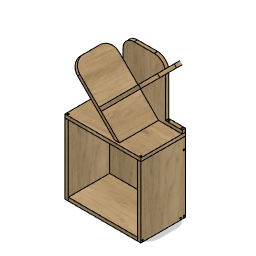
Project 02 Draft 1 (Autodesk Fusion 360 design; units mm, degrees)
Autodesk Fusion 360 part; units mm, degrees
sketch "Sketch1" plane through (0, 0, 0) normal (0, 1, 0) x (1, 0, 0)
  line L0 (0, 0) -> (340, 0)
  line L1 (340, 0) -> (340, -200)
  line L2 (340, -200) -> (0, -200)
  line L3 (0, -200) -> (0, 0)
  line L4 (0, 0) -> (15, 0)
  line L5 (15, 0) -> (15, -200)
  line L6 (15, -200) -> (0, -200)
  line L7 (0, -200) -> (0, 0)
  line L8 (340, 0) -> (325, 0)
  line L9 (325, 0) -> (325, -200)
  line L10 (325, -200) -> (340, -200)
  line L11 (340, -200) -> (340, 0)
  line L12 (15, 0) -> (325, 0)
  line L13 (325, 0) -> (325, -15)
  line L14 (325, -15) -> (15, -15)
  line L15 (15, -15) -> (15, 0)
  dimension "d1" = 340
  dimension "d2" = 200
  dimension "d3" = 15
  dimension "d4" = 15
  dimension "d5" = 15
  constraint horizontal L0
  constraint vertical L1
  constraint horizontal L2
  constraint vertical L3
  constraint coincident L0.start L3.end
  constraint horizontal L4
  constraint vertical L5
  constraint horizontal L6
  constraint vertical L7
  constraint coincident L2 L5.end
  constraint horizontal L8
  constraint vertical L9
  constraint horizontal L10
  constraint vertical L11
  constraint coincident L2 L9.end
  constraint horizontal L12
  constraint vertical L13
  constraint horizontal L14
  constraint vertical L15
  constraint coincident L9 L13.end
  measures "d1" distance of L0.start L0.end
  measures "d2" distance of L0.start L2.end
  measures "d3" distance of L0.start L4.end
  measures "d4" distance of L0.end L8.end
  measures "d5" distance of L4.end L14.end
extrude "Extrude1" add sketch "Sketch1" along normal blind 540 contours L0 L5 L9 L12 L13 L14 L15 makes body 1
extrude "Extrude2" add sketch "Sketch1" along normal blind 540 separate body contours L0 L2 L3 L4 L5 L6 L7 L15 makes body 2
extrude "Extrude3" add sketch "Sketch1" along normal blind 540 separate body contours L0 L1 L2 L8 L9 L10 L11 L13 makes body 3
sketch "Sketch2" plane through (15, 0, 0) normal (1, 0, 0) x (0, 0, -1)
  line L0 (-200, 0) -> (0, 0)
  line L1 (0, 0) -> (0, 540)
  line L2 (0, 540) -> (-200, 540)
  line L3 (-200, 540) -> (-200, 0)
  line L4 (-15, 225) -> (-200, 225)
  line L5 (-200, 225) -> (-200, 240)
  line L6 (-200, 240) -> (-15, 240)
  line L7 (-15, 240) -> (-15, 225)
  dimension "d14" = 15
  constraint horizontal L4
  constraint vertical L5
  constraint horizontal L6
  constraint vertical L7
  constraint coincident L3 L5.end
  measures "d14" distance of L4.start L6.end
extrude "Extrude5" add sketch "Sketch2" along normal blind 310 separate body contours L3 L4 L5 L6 L7 makes body 4
sketch "Sketch3" plane through (0, 540, 0) normal (0, 1, 0) x (-1, 0, 0)
  line L0 (-15, 200) -> (-15, 0)
  line L1 (-15, 0) -> (0, 0)
  line L2 (0, 0) -> (0, 200)
  line L3 (0, 200) -> (-15, 200)
  line L4 (0, 0) -> (-340, 0)
  line L5 (-340, 0) -> (-340, 200)
  line L6 (-340, 200) -> (0, 200)
  line L7 (0, 200) -> (0, 0)
  constraint horizontal L4
  constraint vertical L5
  constraint horizontal L6
  constraint vertical L7
  constraint coincident L1.end L2.start
extrude "Extrude6" add sketch "Sketch3" along normal blind 15 separate body makes body 5
sketch "Sketch4" plane through (0, 555, 0) normal (0, 1, 0) x (-1, 0, 0)
  line L0 (0, 200) -> (-340, 200)
  line L1 (-340, 200) -> (-340, 0)
  line L2 (-340, 0) -> (0, 0)
  line L3 (0, 0) -> (0, 200)
  line L4 (-75, 0) -> (-265, 0)
  line L5 (-265, 0) -> (-265, 15)
  line L6 (-265, 15) -> (-75, 15)
  line L7 (-75, 15) -> (-75, 0)
  dimension "d19" = 15
  constraint horizontal L4
  constraint vertical L5
  constraint horizontal L6
  constraint vertical L7
  constraint coincident L2 L4.start
  measures "d19" distance of L4.start L6.end
extrude "Extrude7" add sketch "Sketch4" along normal blind 250 separate body contours L2 L4 L5 L6 L7 makes body 6
sketch "Sketch5" plane through (0, 0, 15) normal (0, 0, 1) x (1, 0, 0)
  line L0 (75, 555) -> (265, 555)
  line L1 (265, 555) -> (265, 805)
  line L2 (265, 805) -> (75, 805)
  line L3 (75, 805) -> (75, 555)
  line L4 (0, 555) -> (170, 555) construction
  line L5 (170, 555) -> (234, 555) construction
  line L6 (234, 555) -> (21.868, 767.132)
  line L7 (234, 555) -> (494, 555) construction
  line L8 (21.868, 767.132) -> (11.2614, 756.5254)
  line L9 (11.2614, 756.5254) -> (212.7868, 555)
  line L10 (11.2614, 756.5254) -> (284.5456, 756.5254) construction
  line L11 (234, 555) -> (152.6827, 636.3173) construction
  line L12 (152.6827, 636.3173) -> (364.8148, 848.4493)
  line L13 (364.8148, 848.4493) -> (354.2082, 859.0559)
  line L14 (354.2082, 859.0559) -> (142.0761, 646.9239)
  dimension "d22" = 64
  dimension "d23" = 135
  dimension "d24" = 300
  dimension "d25" = 15
  dimension "d26" = 45
  dimension "d27" = 115
  dimension "d28" = 90
  dimension "d29" = 300
  dimension "d30" = 15
  constraint midpoint L0 L4.end
  constraint parallel L0 L4
  constraint coincident L0 L5.end
  constraint horizontal L7
  constraint perpendicular L6 L8
  constraint horizontal L10
  constraint coincident L5 L9.end
  constraint coincident L6 L11.end
  constraint perpendicular L12 L13
  constraint coincident L6 L14.end
  constraint perpendicular L6 L14
  measures "d22" distance of L4.end L5.end
  measures "d23" angle of L6 L7
  measures "d24" distance of L5.end L6.end
  measures "d25" distance of L6.end L8.end
  measures "d26" angle of L9 L10
  measures "d27" distance of L5.end L11.end
  measures "d28" angle of L11 L12
  measures "d29" distance of L11.end L12.end
  measures "d30" distance of L12.end L13.end
extrude "Extrude8" add sketch "Sketch5" along normal blind 175 separate body contours L0 L3 L6 L9 | L3 L6 L8 L9 makes body 7
extrude "Extrude9" add sketch "Sketch5" along normal blind 175 separate body contours L1 L6 L12 L14 | L1 L12 L13 L14 makes body 8
fillet "Fillet1" radius 50 2 edges at (265, 805, 7.5) (75, 805, 7.5) on bodies 6
fillet "Fillet2" radius 50 4 edges at (16.5647, 761.8287, 190) (16.5647, 761.8287, 15) (359.5115, 853.7526, 190) (359.5115, 853.7526, 15) on bodies 7 8
extrude "Extrude10" add 2 faces at (5, 0, 71.6667) (335, 0, 71.6667) along direction (0, -1, 0) blind 90 on bodies 2 3 bodies 2 3 4 5 6 7 8
extrude "Extrude11" add 1 faces at (118.3333, 0, 5) along direction (0, -1, 0) blind 90 on bodies 1 bodies 1
move_body "Move1" bodies 2 3 7 4 5 6 8 1 to x (1, 0, 0) y (0, 1, 0) z (0, 0, 1) at (0, 90, 0)
extrude "Extrude13" cut 1 faces at (118.3333, 0, 5) along direction (0, 1, 0) blind 315 on bodies 1 bodies 1
extrude "Extrude14" cut 1 faces at (5, 0, 66.6667) along direction (0, 1, 0) blind 315 on bodies 2 bodies 2
extrude "Extrude15" cut 1 faces at (330, 0, 66.6667) along direction (0, 1, 0) blind 315 on bodies 3 bodies 3
move_body "Move2" bodies 1 2 5 8 7 6 3 4 to x (1, 0, 0) y (0, 1, 0) z (0, 0, 1) at (0, -315, 0)
sketch "Sketch10" plane through (0, 315, 0) normal (0, 1, 0) x (-1, 0, 0)
  line L0 (-15, 200) -> (-15, 0)
  line L1 (-15, 0) -> (0, 0)
  line L2 (0, 0) -> (0, 200)
  line L3 (0, 200) -> (-15, 200)
  line L4 (0, 0) -> (-7.5, 0) construction
  line L5 (-7.5, 0) -> (-7.5, 7.5) construction
  line L6 (-7.5, 7.5) -> (0, 7.5) construction
  line L7 (0, 7.5) -> (0, 0) construction
  line L8 (0, 200) -> (-7.5, 200) construction
  line L9 (-7.5, 200) -> (-7.5, 192.5) construction
  line L10 (-7.5, 192.5) -> (0, 192.5) construction
  line L11 (0, 192.5) -> (0, 200) construction
  line L12 (-340, 200) -> (-332.5, 200) construction
  line L13 (-332.5, 200) -> (-332.5, 192.5) construction
  line L14 (-332.5, 192.5) -> (-340, 192.5) construction
  line L15 (-340, 192.5) -> (-340, 200) construction
  line L16 (-340, 0) -> (-332.5, 0) construction
  line L17 (-332.5, 0) -> (-332.5, 7.5) construction
  line L18 (-332.5, 7.5) -> (-340, 7.5) construction
  line L19 (-340, 7.5) -> (-340, 0) construction
  circle A0 centre (-7.5, 7.5) radius 4
  circle A1 centre (-7.5, 192.5) radius 4
  circle A2 centre (-332.5, 192.5) radius 4
  circle A3 centre (-332.5, 7.5) radius 4
  dimension "d66" = 7.5
  dimension "d67" = 7.5
  dimension "d68" = 7.5
  dimension "d69" = 7.5
  dimension "d70" = 7.5
  dimension "d71" = 7.5
  dimension "d72" = 7.5
  dimension "d73" = 7.5
  dimension "d74" = 8
  dimension "d75" = 8
  dimension "d76" = 8
  dimension "d77" = 8
  constraint horizontal L4
  constraint vertical L5
  constraint horizontal L6
  constraint vertical L7
  constraint coincident L1.end L2.start
  constraint horizontal L8
  constraint vertical L9
  constraint horizontal L10
  constraint vertical L11
  constraint coincident L2.end L3.start
  constraint horizontal L12
  constraint vertical L13
  constraint horizontal L14
  constraint vertical L15
  constraint horizontal L16
  constraint vertical L17
  constraint horizontal L18
  constraint vertical L19
  constraint coincident L5.end L6.start
  constraint coincident L9.end L10.start
  constraint coincident L13.end L14.start
  constraint coincident L17.end L18.start
  measures "d66" distance of L1.end L4.end
  measures "d67" distance of L1.end L6.end
  measures "d68" distance of L2.end L8.end
  measures "d69" distance of L2.end L10.end
  measures "d70" distance of L12.start L12.end
  measures "d71" distance of L12.start L14.end
  measures "d72" distance of L16.start L16.end
  measures "d73" distance of L16.start L18.end
  measures "d74" diameter of A0
  measures "d75" diameter of A1
  measures "d76" diameter of A2
  measures "d77" diameter of A3
sketch "Sketch11" plane through (265, 0, 0) normal (1, 0, 0) x (0, 0, -1)
  line L0 (0, 530) -> (-15, 530)
  line L1 (-15, 530) -> (-15, 330)
  line L2 (-15, 330) -> (0, 330)
  line L3 (0, 330) -> (0, 530)
  line L4 (-15, 330) -> (0, 330)
  line L5 (0, 330) -> (0, 345)
  line L6 (0, 345) -> (-15, 345)
  line L7 (-15, 345) -> (-15, 330)
  dimension "d78" = 15
  constraint horizontal L4
  constraint vertical L5
  constraint horizontal L6
  constraint vertical L7
  constraint coincident L1.end L2.start
  measures "d78" distance of L1.end L6.end
sketch "Sketch12" plane through (75, 0, 0) normal (-1, 0, 0) x (0, 0, 1)
  line L0 (15, 530) -> (0, 530)
  line L1 (0, 530) -> (0, 330)
  line L2 (0, 330) -> (15, 330)
  line L3 (15, 330) -> (15, 530)
  line L4 (0, 330) -> (15, 330)
  line L5 (15, 330) -> (15, 345)
  line L6 (15, 345) -> (0, 345)
  line L7 (0, 345) -> (0, 330)
  dimension "d79" = 15
  constraint horizontal L4
  constraint vertical L5
  constraint horizontal L6
  constraint vertical L7
  constraint coincident L1.end L2.start
  measures "d79" distance of L1.end L6.end
extrude "Extrude17" add sketch "Sketch12" along normal blind 75 contours L1 L2 L3 L4 L5 L6 L7 bodies 6
extrude "Extrude18" add sketch "Sketch11" along normal blind 75 contours L1 L2 L3 L4 L5 L6 L7 bodies 6
sketch "Sketch20" plane through (340, 0, 0) normal (1, 0, 0) x (0, 0, -1)
  line L0 (-200, 0) -> (0, 0)
  line L1 (0, 0) -> (0, 315)
  line L2 (0, 315) -> (-200, 315)
  line L3 (-200, 315) -> (-200, 0)
  circle A0 centre (-192.5, 7.5) radius 4
  dimension "d99" = 8
  measures "d99" diameter of A0
hole "Hole1" at (340, 7.5, 192.5) direction (-1, 0, 0) diameter 6.78 depth 45 tip angle 118 bodies 3 4
thread "Thread2" "ISO Metric profile 8.0 M8x1.25 6H"
sketch "Sketch21" plane through (0, 0, 190) normal (0, 0, 1) x (1, 0, 0)
  line L0 (57.2233, 506.7767) -> (46.6167, 496.1701)
  line L1 (46.6167, 496.1701) -> (212.7868, 330)
  line L2 (212.7868, 330) -> (234, 330)
  line L3 (234, 330) -> (57.2233, 506.7767)
sketch "Sketch22" plane through (0, 0, 190) normal (0, 0, 1) x (1, 0, 0)
  line L0 (329.4594, 588.094) -> (318.8528, 598.7006)
  line L1 (318.8528, 598.7006) -> (142.0761, 421.9239)
  line L2 (142.0761, 421.9239) -> (152.6827, 411.3173)
  line L3 (152.6827, 411.3173) -> (329.4594, 588.094)
ref_plane "WorkPlane1" through (142.0761, 411.3173, 0) normal (0, 0, 1) x (1, 0, 0)
sketch "Sketch23" plane through (142.0761, 411.3173, 0) normal (0, 0, 1) x (1, 0, 0)
  circle A0 centre (0, 0) radius 4
  circle A1 centre (53.033, -53.033) radius 4
  circle A2 centre (-42.4264, 42.4264) radius 4
  dimension "d106" = 8
  dimension "d107" = 60
  dimension "d108" = 75
  dimension "d109" = 8
  dimension "d110" = 8
  constraint coincident A0.centre origin
  measures "d106" diameter of A0
  measures "d107" distance of A0.centre A2.centre
  measures "d108" distance of A0.centre A1.centre
  measures "d109" diameter of A1
  measures "d110" diameter of A2
sketch "Sketch24" plane through (0, 0, 0) normal (0, 0, -1) x (-1, 0, 0)
  arc A0 (-75, 530) -> (-125, 580) centre (-125, 530) ccw
  line L0 (-125, 580) -> (-215, 580)
  arc A1 (-215, 580) -> (-265, 530) centre (-215, 530) ccw
  line L1 (-265, 530) -> (-265, 345)
  line L2 (-265, 345) -> (-340, 345)
  line L3 (-340, 345) -> (-340, 330)
  line L4 (-340, 330) -> (0, 330)
  line L5 (0, 330) -> (0, 345)
  line L6 (0, 345) -> (-75, 345)
  line L7 (-75, 345) -> (-75, 530)
extrude "Extrude22" cut sketch "Sketch23" along normal blind 45 bodies 6 7
sketch "Sketch25" plane through (0, 0, 190) normal (0, 0, 1) x (1, 0, 0)
ref_plane "WorkPlane2" through (207.4835, 476.7247, 0) normal (0, 0, 1) x (1, 0, 0)
sketch "Sketch26" plane through (207.4835, 476.7247, 0) normal (0, 0, 1) x (1, 0, 0)
  circle A0 centre (0, 0) radius 4
  dimension "d116" = 8
  constraint coincident A0.centre origin
  measures "d116" diameter of A0
extrude "Extrude23" cut sketch "Sketch26" along normal blind 45 bodies 6 8
thread "Thread3" "ISO Metric profile 8.0 M8x1.25 6H" major diameter 8.17 minor diameter 6.7795 pitch 1.25 angle 60 resizes the face on face at (203.5628, 477.5172, 35) on bodies 8
thread "Thread4" "ISO Metric profile 8.0 M8x1.25 6H" major diameter 8.17 minor diameter 6.7795 pitch 1.25 angle 60 resizes the face on face at (203.6072, 477.7117, 5) on bodies 6
thread "Thread5" "ISO Metric profile 8.0 M8x1.25 6H" major diameter 8.17 minor diameter 6.7795 pitch 1.25 angle 60 resizes the face on face at (191.1884, 359.0769, 35) on bodies 7
thread "Thread6" "ISO Metric profile 8.0 M8x1.25 6H" major diameter 8.17 minor diameter 6.7795 pitch 1.25 angle 60 resizes the face on face at (191.2328, 357.2972, 10) on bodies 6
thread "Thread7" "ISO Metric profile 8.0 M8x1.25 6H" major diameter 8.17 minor diameter 6.7795 pitch 1.25 angle 60 resizes the face on face at (138.1998, 410.3303, 35) on bodies 7
thread "Thread8" "ISO Metric profile 8.0 M8x1.25 6H" major diameter 8.17 minor diameter 6.7795 pitch 1.25 angle 60 resizes the face on face at (138.1998, 410.3303, 10) on bodies 6
thread "Thread9" "ISO Metric profile 8.0 M8x1.25 6H" major diameter 8.17 minor diameter 6.7795 pitch 1.25 angle 60 resizes the face on face at (95.7734, 452.7567, 35) on bodies 7
thread "Thread10" "ISO Metric profile 8.0 M8x1.25 6H" major diameter 8.17 minor diameter 6.7795 pitch 1.25 angle 60 resizes the face on face at (95.7734, 452.7567, 10) on bodies 6
sketch "Sketch27" plane through (0, 315, 0) normal (0, 1, 0) x (-1, 0, 0)
extrude "Extrude24" cut sketch "Sketch10" along normal blind 30 contours A0 bodies 5 6
sketch "Sketch28" plane through (0, 345, 0) normal (0, 1, 0) x (-1, 0, 0)
  line L0 (-265, 0) -> (-265, 15)
  line L1 (-265, 15) -> (-340, 15)
  line L2 (-340, 15) -> (-340, 0)
  line L3 (-340, 0) -> (-265, 0)
  line L4 (-340, 7.5) -> (-332.5, 7.5)
  circle A0 centre (-332.5, 7.5) radius 4
  dimension "d121" = 7.5
  dimension "d122" = 8
  constraint midpoint L2 L4.start
  constraint perpendicular L2 L4
  constraint coincident L4.end A0.centre
  measures "d121" distance of L4.start L4.end
  measures "d122" diameter of A0
extrude "Extrude25" cut sketch "Sketch28" against normal blind 60 contours A0 bodies 3 5 6
thread "Thread11" "ISO Metric profile 8.0 M8x1.25 6H" major diameter 8.17 minor diameter 6.7795 pitch 1.25 angle 60 resizes the face on face at (335.1467, 335, 4.5009) on bodies 6
thread "Thread12" "ISO Metric profile 8.0 M8x1.25 6H" major diameter 8.17 minor diameter 6.7795 pitch 1.25 angle 60 resizes the face on face at (335.1467, 320, 4.5009) on bodies 5
thread "Thread13" "ISO Metric profile 8.0 M8x1.25 6H" major diameter 8.17 minor diameter 6.7795 pitch 1.25 angle 60 resizes the face on face at (335.1467, 305, 10.4991) on bodies 3
sketch "Sketch29" plane through (0, 315, 0) normal (0, -1, 0) x (1, 0, 0)
  circle A0 centre (332.5, 7.5) radius 3.3898
  circle A1 centre (7.5, 7.5) radius 4
  line L0 (340, 200) -> (0, 200)
  line L1 (0, 200) -> (0, 0)
  line L2 (0, 0) -> (340, 0)
  line L3 (340, 0) -> (340, 200)
extrude "Extrude26" cut sketch "Sketch29" along normal blind 30 contours A1 bodies 2
thread "Thread14" "ISO Metric profile 8.0 M8x1.25 6H" major diameter 8.17 minor diameter 6.7795 pitch 1.25 angle 60 resizes the face on face at (3.505, 340, 7.6994) on bodies 6
thread "Thread15" "ISO Metric profile 8.0 M8x1.25 6H" major diameter 8.17 minor diameter 6.7795 pitch 1.25 angle 60 resizes the face on face at (3.505, 325, 7.6994) on bodies 5
thread "Thread16" "ISO Metric profile 8.0 M8x1.25 6H" major diameter 8.17 minor diameter 6.7795 pitch 1.25 angle 60 resizes the face on face at (11.4801, 295, 7.1017) on bodies 2
sketch "Sketch30" plane through (0, 345, 0) normal (0, 1, 0) x (-1, 0, 0)
  circle A0 centre (-332.5, 7.5) radius 3.3898
  line L0 (-265, 0) -> (-265, 15)
  line L1 (-265, 15) -> (-340, 15)
  line L2 (-340, 15) -> (-340, 0)
  line L3 (-340, 0) -> (-265, 0)
  line L4 (-265, 7.5) -> (-272.5, 7.5)
  circle A1 centre (-272.5, 7.5) radius 4
  dimension "d127" = 7.5
  dimension "d128" = 8
  constraint midpoint L0 L4.start
  constraint perpendicular L0 L4
  constraint coincident L4.end A1.centre
  measures "d127" distance of L4.start L4.end
  measures "d128" diameter of A1
extrude "Extrude27" cut sketch "Sketch30" against normal blind 60 contours A1 bodies 1 5 6
thread "Thread17" "ISO Metric profile 8.0 M8x1.25 6H" major diameter 8.17 minor diameter 6.7795 pitch 1.25 angle 60 resizes the face on face at (274.3248, 335, 3.9405) on bodies 6
thread "Thread18" "ISO Metric profile 8.0 M8x1.25 6H" major diameter 8.17 minor diameter 6.7795 pitch 1.25 angle 60 resizes the face on face at (274.3248, 320, 3.9405) on bodies 5
thread "Thread19" "ISO Metric profile 8.0 M8x1.25 6H" major diameter 8.17 minor diameter 6.7795 pitch 1.25 angle 60 resizes the face on face at (274.3248, 295, 3.9405) on bodies 1
sketch "Sketch31" plane through (0, 345, 0) normal (0, 1, 0) x (-1, 0, 0)
  circle A0 centre (-7.5, 7.5) radius 3.3898
  line L0 (-75, 15) -> (-75, 0)
  line L1 (-75, 0) -> (0, 0)
  line L2 (0, 0) -> (0, 15)
  line L3 (0, 15) -> (-75, 15)
  line L4 (-75, 7.5) -> (-67.5, 7.5)
  circle A1 centre (-67.5, 7.5) radius 4
  dimension "d131" = 7.5
  dimension "d132" = 8
  constraint midpoint L0 L4.start
  constraint perpendicular L0 L4
  constraint coincident L4.end A1.centre
  measures "d131" distance of L4.start L4.end
  measures "d132" diameter of A1
extrude "Extrude28" cut sketch "Sketch31" against normal blind 60 contours A1 bodies 1 5 6
thread "Thread20" "ISO Metric profile 8.0 M8x1.25 6H" major diameter 8.17 minor diameter 6.7795 pitch 1.25 angle 60 resizes the face on face at (63.5199, 335, 7.1017) on bodies 6
thread "Thread21" "ISO Metric profile 8.0 M8x1.25 6H" major diameter 8.17 minor diameter 6.7795 pitch 1.25 angle 60 resizes the face on face at (63.5199, 320, 7.1017) on face at (63.505, 295, 7.6994) on bodies 1 5
sketch "Sketch32" plane through (0, 0, 0) normal (-1, 0, 0) x (0, 0, 1)
  line L0 (0, 0) -> (200, 0)
  line L1 (200, 0) -> (200, 315)
  line L2 (200, 315) -> (0, 315)
  line L3 (0, 315) -> (0, 0)
hole "Hole2" at (0, 7.5, 192.5) direction (1, 0, 0) diameter 6.78 depth 45 tip angle 118 bodies 2 4
thread "Thread22" "ISO Metric profile 8.0 M8x1.25 6H"
sketch "Sketch33" plane through (0, 0, 0) normal (-1, 0, 0) x (0, 0, 1)
  circle A0 centre (7.5, 7.5) radius 4
  circle A1 centre (22.5, 7.5) radius 4
  dimension "d147" = 8
  dimension "d148" = 8
  measures "d147" diameter of A0
  measures "d148" diameter of A1
hole "Hole3" at (0, 7.5, 7.5) at (0, 7.5, 22.5) direction (1, 0, 0) diameter 6.78 depth 45 tip angle 118 bodies 1 2 4
thread "Thread23" "ISO Metric profile 8.0 M8x1.25 6H"
sketch "Sketch34" plane through (340, 0, 0) normal (1, 0, 0) x (0, 0, -1)
  circle A0 centre (-192.5, 7.5) radius 3.3898
  line L0 (-200, 0) -> (0, 0)
  line L1 (0, 0) -> (0, 315)
  line L2 (0, 315) -> (-200, 315)
  line L3 (-200, 315) -> (-200, 0)
  circle A1 centre (-7.5, 7.5) radius 4
  circle A2 centre (-22.5, 7.5) radius 4
  dimension "d158" = 8
  dimension "d159" = 8
  measures "d158" diameter of A1
  measures "d159" diameter of A2
hole "Hole4" at (340, 7.5, 7.5) at (340, 7.5, 22.5) direction (-1, 0, 0) diameter 6.78 depth 45 tip angle 118 bodies 1 3 4
thread "Thread24" "ISO Metric profile 8.0 M8x1.25 6H"
sketch "Sketch35" plane through (0, 330, 0) normal (0, 1, 0) x (-1, 0, 0)
  circle A0 centre (-67.5, 7.5) radius 3.3898
  circle A1 centre (-272.5, 7.5) radius 3.3898
  circle A2 centre (-332.5, 7.5) radius 3.3898
  circle A3 centre (-7.5, 7.5) radius 3.3898
  line L0 (0, 200) -> (-340, 200)
  line L1 (-340, 200) -> (-340, 0)
  line L2 (-340, 0) -> (0, 0)
  line L3 (0, 0) -> (0, 200)
  line L4 (-340, 200) -> (-332.5, 200)
  line L5 (-340, 192.5) -> (-340, 200)
  circle A4 centre (-332.5, 192.5) radius 4
  constraint horizontal L4
  constraint vertical L5
  constraint coincident L0.end L1.start
extrude "Extrude29" cut sketch "Sketch35" against normal blind 45 contours A4 bodies 3 5
thread "Thread25" "ISO Metric profile 8.0 M8x1.25 6H" major diameter 8.17 minor diameter 6.7795 pitch 1.25 angle 60 resizes the face on face at (329.7071, 325, 195.3635) on bodies 5
sketch "Sketch36" plane through (0, 315, 0) normal (0, -1, 0) x (1, 0, 0)
  circle A0 centre (332.5, 192.5) radius 3.3898
  circle A1 centre (67.5, 7.5) radius 3.3898
  circle A2 centre (272.5, 7.5) radius 3.3898
  circle A3 centre (332.5, 7.5) radius 3.3898
  circle A4 centre (7.5, 7.5) radius 3.3898
  line L0 (340, 200) -> (0, 200)
  line L1 (0, 200) -> (0, 0)
  line L2 (0, 0) -> (340, 0)
  line L3 (340, 0) -> (340, 200)
sketch "Sketch37" plane through (0, 330, 0) normal (0, 1, 0) x (-1, 0, 0)
  circle A0 centre (-332.5, 192.5) radius 3.3898
  circle A1 centre (-67.5, 7.5) radius 3.3898
  circle A2 centre (-272.5, 7.5) radius 3.3898
  circle A3 centre (-332.5, 7.5) radius 3.3898
  circle A4 centre (-7.5, 7.5) radius 3.3898
  line L0 (0, 200) -> (-340, 200)
  line L1 (-340, 200) -> (-340, 0)
  line L2 (-340, 0) -> (0, 0)
  line L3 (0, 0) -> (0, 200)
  line L4 (0, 200) -> (-7.5, 200)
  line L5 (0, 192.5) -> (0, 200)
  circle A5 centre (-7.5, 192.5) radius 4
  dimension "d170" = 8
  constraint horizontal L4
  constraint vertical L5
  constraint coincident L0.start L3.end
  measures "d170" diameter of A5
extrude "Extrude30" cut sketch "Sketch37" against normal blind 45 contours A5 bodies 2 5
thread "Thread26" "ISO Metric profile 8.0 M8x1.25 6H" major diameter 8.17 minor diameter 6.7795 pitch 1.25 angle 60 resizes the face on face at (11.1859, 320, 190.9463) on bodies 5
sketch "Sketch38" plane through (0, 330, 0) normal (0, 1, 0) x (-1, 0, 0)
  circle A0 centre (-7.5, 192.5) radius 3.3898
  circle A1 centre (-332.5, 192.5) radius 3.3898
  circle A2 centre (-67.5, 7.5) radius 3.3898
  circle A3 centre (-272.5, 7.5) radius 3.3898
  circle A4 centre (-332.5, 7.5) radius 3.3898
  circle A5 centre (-7.5, 7.5) radius 3.3898
  line L0 (0, 200) -> (-340, 200)
  line L1 (-340, 200) -> (-340, 0)
  line L2 (-340, 0) -> (0, 0)
  line L3 (0, 0) -> (0, 200)
sketch "Sketch39" plane through (0, 0, 190) normal (0, 0, 1) x (1, 0, 0)
sketch "Sketch40" plane through (0, 315, 0) normal (0, -1, 0) x (1, 0, 0)
sketch "Sketch41" plane through (0, 0, 200) normal (0, 0, 1) x (1, 0, 0)
  line L0 (0, 315) -> (340, 315)
  line L1 (340, 315) -> (340, 330)
  line L2 (340, 330) -> (0, 330)
  line L3 (0, 330) -> (0, 315)
sketch "Sketch42" plane through (0, 330, 0) normal (0, 1, 0) x (-1, 0, 0)
sketch "Sketch43" plane through (0, 315, 0) normal (0, -1, 0) x (1, 0, 0)
sketch "Sketch44" plane through (170, 315, 100) normal (0, -1, 0) x (1, 0, 0)
sketch "Sketch45" plane through (0, 315, 0) normal (0, -1, 0) x (1, 0, 0)
  line L0 (0, 200) -> (0, 190)
  line L1 (0, 190) -> (223.4627, 185.9165)
  line L2 (223.4627, 185.9165) -> (223.0973, 165.9199)
  circle A0 centre (223.0973, 165.9199) radius 4
  dimension "d173" = 223.5
  dimension "d174" = 20
  dimension "d175" = 8
  constraint vertical L0
  constraint perpendicular L1 L2
  constraint coincident L2.end A0.centre
  measures "d173" distance of L0.end L1.end
  measures "d174" distance of L1.end L2.end
  measures "d175" diameter of A0
extrude "Extrude31" cut sketch "Sketch45" against normal blind 17.5 bodies 5 7
thread "Thread27" "ISO Metric profile 8.0 M8x1.25 6H" major diameter 8.17 minor diameter 6.7795 pitch 1.25 angle 60 resizes the face on face at (226.6102, 325, 167.8329) on bodies 5
sketch "Sketch46" plane through (0, 315, 0) normal (0, -1, 0) x (1, 0, 0)
sketch "Sketch47" plane through (0, 345, 0) normal (0, 1, 0) x (-1, 0, 0)
  circle A0 centre (-272.5, 7.5) radius 3.3898
  circle A1 centre (-332.5, 7.5) radius 3.3898
  line L0 (-265, 0) -> (-265, 15)
  line L1 (-265, 15) -> (-340, 15)
  line L2 (-340, 15) -> (-340, 0)
  line L3 (-340, 0) -> (-265, 0)
sketch "Sketch48" plane through (0, 315, 0) normal (0, -1, 0) x (1, 0, 0)
  line L0 (223, 162) -> (223, 20)
  circle A0 centre (223, 20) radius 4
  dimension "d178" = 142
  dimension "d179" = 8
  constraint vertical L0
  constraint coincident L0.end A0.centre
  measures "d178" distance of L0.start L0.end
  measures "d179" diameter of A0
extrude "Extrude32" cut sketch "Sketch48" against normal blind 17.5 bodies 5 7
thread "Thread28" "ISO Metric profile 8.0 M8x1.25 6H" major diameter 8.17 minor diameter 6.7795 pitch 1.25 angle 60 resizes the face on face at (219.9358, 320, 22.5712) on bodies 5
thread "Thread29" "ISO Metric profile 8.0 M8x1.25 6H" major diameter 8.17 minor diameter 6.7795 pitch 1.25 angle 60 resizes the face on face at (219.6841, 331.6667, 163.8341) on bodies 7
thread "Thread30" "ISO Metric profile 8.0 M8x1.25 6H" major diameter 8.17 minor diameter 6.7795 pitch 1.25 angle 60 resizes the face on face at (219.9358, 331.6667, 17.4289) on bodies 7
sketch "Sketch49" plane through (340, 0, 0) normal (1, 0, 0) x (0, 0, -1)
  circle A0 centre (-7.5, 7.5) radius 3.3898
  circle A1 centre (-22.5, 7.5) radius 3.3898
  circle A2 centre (-192.5, 7.5) radius 3.3898
  line L0 (-200, 0) -> (0, 0)
  line L1 (0, 0) -> (0, 315)
  line L2 (0, 315) -> (-200, 315)
  line L3 (-200, 315) -> (-200, 0)
  line L4 (0, 315) -> (-7.5, 315) construction
  line L5 (-7.5, 315) -> (-7.5, 265) construction
  line L6 (-7.5, 265) -> (0, 265) construction
  line L7 (0, 265) -> (0, 315) construction
  circle A3 centre (-7.5, 265) radius 4
  dimension "d182" = 7.5
  dimension "d183" = 50
  dimension "d184" = 8
  constraint horizontal L4
  constraint vertical L5
  constraint horizontal L6
  constraint vertical L7
  constraint coincident L1.end L2.start
  constraint coincident L5.end L6.start
  measures "d182" distance of L1.end L4.end
  measures "d183" distance of L1.end L6.end
  measures "d184" diameter of A3
sketch "Sketch50" plane through (0, 0, 0) normal (-1, 0, 0) x (0, 0, 1)
  circle A0 centre (7.5, 7.5) radius 3.3898
  circle A1 centre (22.5, 7.5) radius 3.3898
  circle A2 centre (192.5, 7.5) radius 3.3898
  line L0 (0, 0) -> (200, 0)
  line L1 (200, 0) -> (200, 315)
  line L2 (200, 315) -> (0, 315)
  line L3 (0, 315) -> (0, 0)
  line L4 (0, 315) -> (7.5, 315) construction
  line L5 (7.5, 315) -> (7.5, 265) construction
  line L6 (7.5, 265) -> (0, 265) construction
  line L7 (0, 265) -> (0, 315) construction
  circle A3 centre (7.5, 265) radius 4
  dimension "d185" = 7.5
  dimension "d186" = 50
  dimension "d187" = 8
  constraint horizontal L4
  constraint vertical L5
  constraint horizontal L6
  constraint vertical L7
  constraint coincident L2.end L3.start
  constraint coincident L5.end L6.start
  measures "d185" distance of L2.end L4.end
  measures "d186" distance of L2.end L6.end
  measures "d187" diameter of A3
extrude "Extrude33" cut sketch "Sketch50" against normal blind 15 contours A3 bodies 2
extrude "Extrude34" cut sketch "Sketch49" against normal blind 15 contours A3 bodies 3
extrude "Extrude35" cut sketch "Sketch49" against normal blind 45 contours A3 bodies 1
extrude "Extrude36" cut sketch "Sketch50" against normal blind 45 contours A3 bodies 1
thread "Thread31" "ISO Metric profile 8.0 M8x1.25 6H" major diameter 8.17 minor diameter 6.7795 pitch 1.25 angle 60 resizes the face on face at (305, 265.987, 3.6237) on face at (35, 265.7926, 3.5793) on bodies 1
thread "Thread32" "ISO Metric profile 8.0 M8x1.25 6H" major diameter 8.17 minor diameter 6.7795 pitch 1.25 angle 60 resizes the face on face at (330, 265.987, 3.6237) on face at (10, 265.7926, 3.5793) on bodies 2 3
sketch "Sketch51" plane through (0, 0, 0) normal (0, 0, -1) x (-1, 0, 0)
  line L0 (-325, 0) -> (-15, 0)
  line L1 (-15, 0) -> (-15, 315)
  line L2 (-15, 315) -> (-325, 315)
  line L3 (-325, 315) -> (-325, 0)
  line L4 (-15, 0) -> (-65, 0) construction
  line L5 (-65, 0) -> (-65, 7.5) construction
  line L6 (-65, 7.5) -> (-15, 7.5) construction
  line L7 (-15, 7.5) -> (-15, 0) construction
  line L8 (-325, 0) -> (-275, 0) construction
  line L9 (-275, 0) -> (-275, 7.5) construction
  line L10 (-275, 7.5) -> (-325, 7.5) construction
  line L11 (-325, 7.5) -> (-325, 0) construction
  circle A0 centre (-275, 7.5) radius 4
  circle A1 centre (-65, 7.5) radius 4
  dimension "d196" = 50
  dimension "d197" = 7.5
  dimension "d198" = 50
  dimension "d199" = 7.5
  dimension "d200" = 8
  dimension "d201" = 8
  constraint horizontal L4
  constraint vertical L5
  constraint horizontal L6
  constraint vertical L7
  constraint coincident L0.end L1.start
  constraint horizontal L8
  constraint vertical L9
  constraint horizontal L10
  constraint vertical L11
  constraint coincident L0.start L3.end
  constraint coincident L9.end L10.start
  constraint coincident L5.end L6.start
  measures "d196" distance of L0.end L4.end
  measures "d197" distance of L0.end L6.end
  measures "d198" distance of L0.start L8.end
  measures "d199" distance of L0.start L10.end
  measures "d200" diameter of A0
  measures "d201" diameter of A1
extrude "Extrude37" cut sketch "Sketch51" against normal blind 15 contours A0 | A1 bodies 1
thread "Thread33" "ISO Metric profile 8.0 M8x1.25 6H" major diameter 8.17 minor diameter 6.7795 pitch 1.25 angle 60 resizes the face on face at (277.7929, 10.3635, 10) on face at (61.0199, 7.1017, 10) on bodies 1
extrude "Extrude38" cut sketch "Sketch51" against normal blind 45 contours A0 | A1 bodies 4
thread "Thread34" "ISO Metric profile 8.0 M8x1.25 6H" major diameter 8.17 minor diameter 6.7795 pitch 1.25 angle 60 resizes the face on face at (61.0199, 7.1017, 35) on face at (277.6467, 10.4991, 25) on bodies 4
sketch "Sketch52" plane through (282, 282, 0) normal (-0.707107, -0.707107, 0) x (0, 0, 1)
  line L0 (15, 197.8823) -> (15, 182.8823)
  line L1 (15, 182.8823) -> (190, 182.8823)
  line L2 (190, 182.8823) -> (190, 197.8823)
  line L3 (190, 197.8823) -> (15, 197.8823)
  circle A0 centre (182.5, 190.3823) radius 4
  circle A1 centre (58.5, 190.3823) radius 4
  dimension "d208" = 8
  dimension "d210" = 8
  measures "d208" diameter of A0
  measures "d210" diameter of A1
extrude "Extrude39" cut sketch "Sketch52" along normal blind 40 contours A0 | A1 bodies 7
extrude "Extrude40" cut sketch "Sketch52" against normal blind 30 contours A0 | A1 bodies 8
thread "Thread35" "ISO Metric profile 8.0 M8x1.25 6H" major diameter 8.17 minor diameter 6.7795 pitch 1.25 angle 60 resizes the face on face at (160.8236, 431.4607, 62.3763) on face at (162.082, 430.2023, 178.5793) on bodies 8
thread "Thread36" "ISO Metric profile 8.0 M8x1.25 6H" major diameter 8.17 minor diameter 6.7795 pitch 1.25 angle 60 resizes the face on face at (143.2834, 413.6455, 62.4207) on face at (144.5418, 412.3871, 178.6237) on bodies 7
named bodies: "หลัง", "ซ้าย", "ฐาน", "บนแปลก", "เอียงซ้าย", "เอียงขวา", "ขวา"
